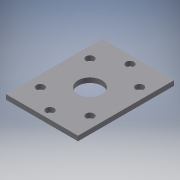
# Autodesk Inventor part: XMotorMount
Saved by Autodesk Inventor 2019 (Build 230136000, 136)
## iProperties
Created: 2019-08-19
Part Number: XMotorMount
Material: Generic
Document SubType Name: Modeling
Designer: Bruno
Density: 1 g/cm^3
Appearance: Default
Author: Bruno
Autodesk Inventor part; units mm, degrees
ref_plane "YZ Plane" through (0, 0, 0) normal (1, 0, 0) x (0, 1, 0)
ref_plane "XZ Plane" through (0, 0, 0) normal (0, 1, 0) x (-1, 0, 0)
ref_plane "XY Plane" through (0, 0, 0) normal (0, 0, 1) x (1, 0, 0)
sketch "Sketch1" plane through (0, 0, 0) normal (0, 1, 0) x (-1, 0, 0)
  line L0 (22.5, -30) -> (-22.5, -30)
  line L1 (-22.5, -30) -> (-22.5, 30)
  line L2 (-22.5, 30) -> (22.5, 30)
  line L3 (22.5, 30) -> (22.5, -30)
  line L4 (0, 0) -> (0, -2.1911) construction
  line L5 (0, 0) -> (-2.34, 0) construction
  line L6 (15.5, -15.5) -> (-15.5, -15.5) construction
  line L7 (-15.5, -15.5) -> (-15.5, 15.5) construction
  line L8 (-15.5, 15.5) -> (15.5, 15.5) construction
  line L9 (15.5, 15.5) -> (15.5, -15.5) construction
  circle A0 centre (15.5, -15.5) radius 2.5
  circle A1 centre (-15.5, -15.5) radius 2.5
  circle A2 centre (-15.5, 15.5) radius 2.5
  circle A3 centre (15.5, 15.5) radius 2.5
  circle A4 centre (0, -25) radius 2.5
  circle A5 centre (0, 25) radius 2.5
  line L10 (0, -25) -> (0, -30) construction
  line L11 (0, 30) -> (0, 25) construction
  circle A6 centre (0, 0) radius 7.5
  point P0 (0, -1.0955)
  dimension "d6" = 60
  dimension "d7" = 45
  dimension "d8" = 31
  dimension "d9" = 5
  dimension "d10" = 5
  dimension "d11" = 5
  dimension "d12" = 5
  dimension "d13" = 5
  dimension "d14" = 5
  dimension "d15" = 15
  constraints: 24 end point, 7 centre point, 5 coincident, 4 horizontal, 4 parallel, 3 midpoint, 3 vertical, 2 equal length, 2 perpendicular, 1 equal radius, 5 other
  measures "d6" distance of L0.end L1.end
  measures "d7" distance of L1.end L2.end
  measures "d8" distance of L6.end L7.end
  measures "d9" diameter of A0
  measures "d10" diameter of A1
  measures "d11" diameter of A2
  measures "d12" diameter of A3
  measures "d13" diameter of A4
  measures "d14" distance from line of L0 L10.start
  measures "d15" diameter of A6
extrude "Extrusion1" add sketch "Sketch1" along normal blind 3
body "Solid1"
